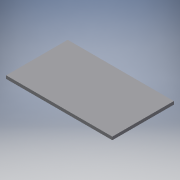
# Autodesk Inventor part: Onderkant
Saved by Autodesk Inventor 2018.3 (Build 223284000, 284)
## iProperties
Created: 2020-11-10
Part Number: Onderkant
Material: Generic
Document SubType Name: Modeling
Designer: daanv
Density: 1 g/cm^3
Appearance: Default
Author: daanv
Autodesk Inventor part; units mm, degrees
ref_plane "YZ Plane" through (0, 0, 0) normal (1, 0, 0) x (0, 1, 0)
ref_plane "XZ Plane" through (0, 0, 0) normal (0, 1, 0) x (-1, 0, 0)
ref_plane "XY Plane" through (0, 0, 0) normal (0, 0, 1) x (1, 0, 0)
sketch "Sketch1" plane through (0, 0, 0) normal (0, 0, 1) x (1, 0, 0)
  line L0 (0, 0) -> (34.5, 0)
  line L1 (34.5, 0) -> (34.5, 20)
  line L2 (34.5, 20) -> (0, 20)
  line L3 (0, 20) -> (0, 0)
  dimension "d0" = 34.5
  dimension "d1" = 20
  constraints: 8 end point, 2 parallel, 1 horizontal, 1 perpendicular
  measures "d0" distance of L2.end L1.end
  measures "d1" distance of L1.end L0.end
extrude "Extrusion1" add sketch "Sketch1" along normal blind 1
body "Solid1"
